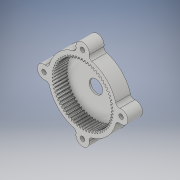
# Autodesk Inventor part: RushGears_AP214_F3264A
Saved by Autodesk Inventor 2019 (Build 230136000, 136)
## iProperties
Company: Microsoft
Created: 2015-06-23
Part Number: RushGears_AP214_F3264A
Material: Generic
Description: STEP AP214
Document SubType Name: Modeling
Designer: test
Density: 1 g/cm^3
Appearance: Default
Sending System: SolidWorks 2010
Preprocessor: SwSTEP 2.0
Title: 698691a11791bb78f6e835ded6c04318_ap214.step
Author: Solidworks
Revision Number: ANY
Autodesk Inventor part; units mm, degrees
(part 1 of 4)
ref_plane "YZ Plane" through (0, 0, 0) normal (1, 0, 0) x (0, 1, 0)
ref_plane "Work Plane2" through (20.4322, -12.3376, 4.826) normal (0, 0, 1) x (0.8768168, -0.4808246, 0)
ref_plane "Work Plane1" through (20.4322, -12.3376, 27.051) normal (0, 0, 1) x (0.8768168, -0.4808246, 0)
sketch "Sketch2" plane through (20.4322, -12.3376, 27.051) normal (0, 0, 1) x (0.8768168, -0.4808246, 0)
  arc A0 (1.0525, 9.1239) -> (0.8407, 9.7461) centre (-23.8475, 0.9936) ccw projected
  arc A1 (0.8407, 9.7461) -> (-0.8407, 9.7461) centre (0, 0) ccw projected
  arc A2 (-1.1493, 9.9373) -> (-0.8407, 9.7461) centre (-0.8668, 10.0487) ccw projected
  arc A3 (-1.1493, 9.9373) -> (-1.1833, 10.0231) centre (-23.8475, 0.9936) ccw projected
  arc A4 (-1.0894, 10.3738) -> (-1.1833, 10.0231) centre (-0.9012, 10.1355) ccw projected
  arc A5 (-1.0894, 10.3738) -> (0.1357, 11.5254) centre (-7.1521, 18.0509) ccw projected
  arc A6 (0.1357, 11.5254) -> (-0.1361, 12.1238) centre (-23.8475, 0.9936) ccw projected
  arc A7 (-0.1361, 12.1238) -> (-1.8093, 11.959) centre (-0.0174, 2.3422) ccw projected
  arc A8 (-2.1353, 12.1191) -> (-1.8093, 11.959) centre (-1.865, 12.2576) ccw projected
  arc A9 (-2.1353, 12.1191) -> (-2.1775, 12.2011) centre (-23.8475, 0.9936) ccw projected
  arc A10 (-2.1184, 12.5594) -> (-2.1775, 12.2011) centre (-1.9077, 12.3406) ccw projected
  arc A11 (-2.1184, 12.5594) -> (-1.0121, 13.8254) centre (-8.9044, 19.6052) ccw projected
  arc A12 (-1.0121, 13.8254) -> (-1.3412, 14.3943) centre (-23.8475, 0.9936) ccw projected
  arc A13 (-1.3412, 14.3943) -> (-2.9903, 14.0663) centre (-0.2644, 4.6715) ccw projected
  arc A14 (-3.3303, 14.1937) -> (-2.9903, 14.0663) centre (-3.0749, 14.358) ccw projected
  arc A15 (-3.3303, 14.1937) -> (-3.3804, 14.2712) centre (-23.8475, 0.9936) ccw projected
  arc A16 (-3.3567, 14.6335) -> (-3.3804, 14.2712) centre (-3.1256, 14.4365) ccw projected
  arc A17 (-3.3567, 14.6335) -> (-2.3798, 16.0019) centre (-10.8006, 20.9803) ccw projected
  arc A18 (-2.3798, 16.0019) -> (-2.7631, 16.5358) centre (-23.8475, 0.9936) ccw projected
  arc A19 (-2.7631, 16.5358) -> (-4.3721, 16.0477) centre (-0.7385, 6.9653) ccw projected
  arc A20 (-4.7229, 16.1411) -> (-4.3721, 16.0477) centre (-4.4849, 16.3297) ccw projected
  arc A21 (-4.7229, 16.1411) -> (-4.7804, 16.2134) centre (-23.8475, 0.9936) ccw projected
  arc A22 (-4.7923, 16.5763) -> (-4.7804, 16.2134) centre (-4.543, 16.4028) ccw projected
  arc A23 (-4.7923, 16.5763) -> (-3.9543, 18.0339) centre (-12.8224, 22.1628) ccw projected
  arc A24 (-3.9543, 18.0339) -> (-4.3881, 18.5276) centre (-23.8475, 0.9936) ccw projected
  arc A25 (-4.3881, 18.5276) -> (-5.9414, 17.8842) centre (-1.4351, 9.2017) ccw projected
  arc A26 (-6.2997, 17.9427) -> (-5.9414, 17.8842) centre (-6.0813, 18.1537) ccw projected
  arc A27 (-6.2997, 17.9427) -> (-6.364, 18.009) centre (-23.8475, 0.9936) ccw projected
  arc A28 (-6.4114, 18.369) -> (-6.364, 18.009) centre (-6.1463, 18.2208) ccw projected
  arc A29 (-6.4114, 18.369) -> (-5.7203, 19.9017) centre (-14.9505, 23.1415) ccw projected
  arc A30 (-5.7203, 19.9017) -> (-6.2004, 20.3505) centre (-23.8475, 0.9936) ccw projected
  arc A31 (-6.2004, 20.3505) -> (-7.6832, 19.5579) centre (-2.3475, 11.359) ccw projected
  arc A32 (-8.0455, 19.5811) -> (-7.6832, 19.5579) centre (-7.8488, 19.8125) ccw projected
  arc A33 (-8.0455, 19.5811) -> (-8.116, 19.6407) centre (-23.8475, 0.9936) ccw projected
  arc A34 (-8.1985, 19.9943) -> (-8.116, 19.6407) centre (-7.9201, 19.8729) ccw projected
  arc A35 (-8.1985, 19.9943) -> (-7.6609, 21.5874) centre (-17.1642, 23.907) ccw projected
  arc A36 (-7.6609, 21.5874) -> (-8.1827, 21.987) centre (-23.8475, 0.9936) ccw projected
  arc A37 (-8.1827, 21.987) -> (-9.5807, 21.0529) centre (-3.467, 13.4164) ccw projected
  arc A38 (-9.9435, 21.0405) -> (-9.5807, 21.0529) centre (-9.7705, 21.29) ccw projected
  arc A39 (-9.9435, 21.0405) -> (-10.0195, 21.0929) centre (-23.8475, 0.9936) ccw projected
  arc A40 (-10.1362, 21.4367) -> (-10.0195, 21.0929) centre (-9.8473, 21.3431) ccw projected
  arc A41 (-10.1362, 21.4367) -> (-9.7574, 23.0748) centre (-19.4423, 24.4517) ccw projected
  arc A42 (-9.7574, 23.0748) -> (-10.3158, 23.4214) centre (-23.8475, 0.9936) ccw projected
  arc A43 (-10.3158, 23.4214) -> (-11.6155, 22.3547) centre (-4.7828, 15.3542) ccw projected
  arc A44 (-11.9754, 22.3068) -> (-11.6155, 22.3547) centre (-11.8276, 22.5721) ccw projected
  arc A45 (-11.9754, 22.3068) -> (-12.0561, 22.3515) centre (-23.8475, 0.9936) ccw projected
  arc A46 (-12.206, 22.6822) -> (-12.0561, 22.3515) centre (-11.9093, 22.6174) ccw projected
  arc A47 (-12.206, 22.6822) -> (-11.9896, 24.3495) centre (-21.7628, 24.7705) ccw projected
  arc A48 (-11.9896, 24.3495) -> (-12.5793, 24.6397) centre (-23.8475, 0.9936) ccw projected
  arc A49 (-12.5793, 24.6397) -> (-13.7682, 23.4508) centre (-6.2822, 17.1537) ccw projected
  arc A50 (-14.1217, 23.3678) -> (-13.7682, 23.4508) centre (-14.0006, 23.6463) ccw projected
  arc A51 (-14.1217, 23.3678) -> (-14.2064, 23.4044) centre (-23.8475, 0.9936) ccw projected
  arc A52 (-14.388, 23.7188) -> (-14.2064, 23.4044) centre (-14.0863, 23.6834) ccw projected
  arc A53 (-14.388, 23.7188) -> (-14.336, 25.3994) centre (-24.1034, 24.8604) ccw projected
  arc A54 (-14.336, 25.3994) -> (-14.9513, 25.6303) centre (-23.8475, 0.9936) ccw projected
  arc A55 (-14.9513, 25.6303) -> (-16.0179, 24.3306) centre (-7.9508, 18.7976) ccw projected
  arc A56 (-16.3615, 24.2134) -> (-16.0179, 24.3306) centre (-16.2684, 24.5024) ccw projected
  arc A57 (-16.3615, 24.2134) -> (-16.4494, 24.2415) centre (-23.8475, 0.9936) ccw projected
  arc A58 (-16.661, 24.5366) -> (-16.4494, 24.2415) centre (-16.3573, 24.5309) ccw projected
  arc A59 (-16.661, 24.5366) -> (-16.774, 26.2141) centre (-26.4415, 24.7204) ccw projected
  arc A60 (-16.774, 26.2141) -> (-17.409, 26.3837) centre (-23.8475, 0.9936) ccw projected
  arc A61 (-17.409, 26.3837) -> (-18.3431, 24.9857) centre (-9.7724, 20.27) ccw projected
  arc A62 (-18.6735, 24.8353) -> (-18.3431, 24.9857) centre (-18.6091, 25.1321) ccw projected
  arc A63 (-18.6735, 24.8353) -> (-18.7637, 24.8547) centre (-23.8475, 0.9936) ccw projected
  arc A64 (-19.0032, 25.1276) -> (-18.7637, 24.8547) centre (-18.7005, 25.1517) ccw projected
  arc A65 (-19.0032, 25.1276) -> (-19.2801, 26.786) centre (-28.7547, 24.3519) ccw projected
  arc A66 (-19.2801, 26.786) -> (-19.9286, 26.8925) centre (-23.8475, 0.9936) ccw projected
  arc A67 (-19.9286, 26.8925) -> (-20.7212, 25.4097) centre (-11.7296, 21.5568) ccw projected
  arc A68 (-21.0353, 25.2276) -> (-20.7212, 25.4097) centre (-21.0003, 25.5293) ccw projected
  arc A69 (-21.0353, 25.2276) -> (-21.127, 25.2381) centre (-23.8475, 0.9936) ccw projected
  arc A70 (-21.3921, 25.4863) -> (-21.127, 25.2381) centre (-21.0932, 25.5399) ccw projected
  arc A71 (-21.3921, 25.4863) -> (-21.8302, 27.1095) centre (-31.0205, 23.7584) ccw projected
  arc A72 (-21.8302, 27.1095) -> (-22.486, 27.1519) centre (-23.8475, 0.9936) ccw projected
  arc A73 (-22.486, 27.1519) -> (-23.1295, 25.5986) centre (-13.8035, 22.6456) ccw projected
  arc A74 (-23.4242, 25.3866) -> (-23.1295, 25.5986) centre (-23.419, 25.6902) ccw projected
  arc A75 (-23.4242, 25.3866) -> (-23.5165, 25.388) centre (-23.8475, 0.9936) ccw projected
  arc A76 (-23.8046, 25.609) -> (-23.5165, 25.388) centre (-23.5124, 25.6917) ccw projected
  arc A77 (-23.8046, 25.609) -> (-24.3997, 27.1815) centre (-33.2174, 22.9457) ccw projected
  arc A78 (-24.3997, 27.1815) -> (-25.0566, 27.1594) centre (-23.8475, 0.9936) ccw projected
  arc A79 (-25.0566, 27.1594) -> (-25.5446, 25.5505) centre (-15.9742, 23.5258) ccw projected
  arc A80 (-25.8172, 25.3106) -> (-25.5446, 25.5505) centre (-25.8417, 25.6133) ccw projected
  arc A81 (-25.8172, 25.3106) -> (-25.9092, 25.303) centre (-23.8475, 0.9936) ccw projected
  arc A82 (-26.2175, 25.4947) -> (-25.9092, 25.303) centre (-25.9348, 25.6056) ccw projected
  arc A83 (-26.2175, 25.4947) -> (-26.9639, 27.0013) centre (-35.3239, 21.9216) ccw projected
  arc A84 (-26.9639, 27.0013) -> (-27.6154, 26.9149) centre (-23.8475, 0.9936) ccw projected
  arc A85 (-27.6154, 26.9149) -> (-27.9434, 25.2659) centre (-18.2206, 24.189) ccw projected
  arc A86 (-28.1912, 25.0005) -> (-27.9434, 25.2659) centre (-28.2453, 25.2993) ccw projected
  arc A87 (-28.1912, 25.0005) -> (-28.282, 24.9839) centre (-23.8475, 0.9936) ccw projected
  arc A88 (-28.6077, 25.1444) -> (-28.282, 24.9839) centre (-28.3372, 25.2825) ccw projected
  arc A89 (-28.6077, 25.1444) -> (-29.4981, 26.5706) centre (-37.32, 20.6959) ccw projected
  arc A90 (-29.4981, 26.5706) -> (-30.138, 26.4207) centre (-23.8475, 0.9936) ccw projected
  arc A91 (-30.138, 26.4207) -> (-30.3028, 24.7475) centre (-20.5213, 24.6288) ccw projected
  arc A92 (-30.5234, 24.4591) -> (-30.3028, 24.7475) centre (-30.6065, 24.7512) ccw projected
  arc A93 (-30.5234, 24.4591) -> (-30.6121, 24.4337) centre (-23.8475, 0.9936) ccw projected
  arc A94 (-30.9519, 24.5615) -> (-30.6121, 24.4337) centre (-30.6963, 24.7255) ccw projected
  arc A95 (-30.9519, 24.5615) -> (-31.9779, 25.8935) centre (-39.1863, 19.2805) ccw projected
  arc A96 (-31.9779, 25.8935) -> (-32.6, 25.6817) centre (-23.8475, 0.9936) ccw projected
  arc A97 (-32.6, 25.6817) -> (-32.6, 24.0004) centre (-22.8539, 24.8411) ccw projected
  arc A98 (-32.7913, 23.6917) -> (-32.6, 24.0004) centre (-32.9026, 23.9743) ccw projected
  arc A99 (-32.7913, 23.6917) -> (-32.8771, 23.6578) centre (-23.8475, 0.9936) ccw projected
  arc A100 (-33.2278, 23.7517) -> (-32.8771, 23.6578) centre (-32.9895, 23.9399) ccw projected
  arc A101 (-33.2278, 23.7517) -> (-34.3794, 24.9767) centre (-40.9048, 17.689) ccw projected
  arc A102 (-34.3794, 24.9767) -> (-34.9778, 24.7049) centre (-23.8475, 0.9936) ccw projected
  arc A103 (-34.9778, 24.7049) -> (-34.813, 23.0317) centre (-25.1962, 24.8236) ccw projected
  arc A104 (-34.973, 22.7058) -> (-34.813, 23.0317) centre (-35.1115, 22.9761) ccw projected
  arc A105 (-34.973, 22.7058) -> (-35.0551, 22.6636) centre (-23.8475, 0.9936) ccw projected
  arc A106 (-35.4133, 22.7227) -> (-35.0551, 22.6636) centre (-35.1946, 22.9333) ccw projected
  arc A107 (-35.4133, 22.7227) -> (-36.6794, 23.8289) centre (-42.4591, 15.9367) ccw projected
  arc A108 (-36.6794, 23.8289) -> (-37.2483, 23.4998) centre (-23.8475, 0.9936) ccw projected
  arc A109 (-37.2483, 23.4998) -> (-36.9203, 21.8508) centre (-27.5255, 24.5767) ccw projected
  arc A110 (-37.0476, 21.5108) -> (-36.9203, 21.8508) centre (-37.2119, 21.7662) ccw projected
  arc A111 (-37.0476, 21.5108) -> (-37.1251, 21.4607) centre (-23.8475, 0.9936) ccw projected
  arc A112 (-37.4874, 21.4844) -> (-37.1251, 21.4607) centre (-37.2904, 21.7155) ccw projected
  arc A113 (-37.4874, 21.4844) -> (-38.8559, 22.4612) centre (-43.8342, 14.0405) ccw projected
  arc A114 (-38.8559, 22.4612) -> (-39.3898, 22.0779) centre (-23.8475, 0.9936) ccw projected
  arc A115 (-39.3898, 22.0779) -> (-38.9017, 20.469) centre (-29.8193, 24.1026) ccw projected
  arc A116 (-38.9951, 20.1181) -> (-38.9017, 20.469) centre (-39.1836, 20.3562) ccw projected
  arc A117 (-38.9951, 20.1181) -> (-39.0673, 20.0607) centre (-23.8475, 0.9936) ccw projected
  arc A118 (-39.4302, 20.0488) -> (-39.0673, 20.0607) centre (-39.2568, 20.2981) ccw projected
  arc A119 (-39.4302, 20.0488) -> (-40.8878, 20.8868) centre (-45.0168, 12.0186) ccw projected
  arc A120 (-40.8878, 20.8868) -> (-41.3815, 20.453) centre (-23.8475, 0.9936) ccw projected
  arc A121 (-41.3815, 20.453) -> (-40.7381, 18.8997) centre (-32.0556, 23.406) ccw projected
  arc A122 (-40.7967, 18.5413) -> (-40.7381, 18.8997) centre (-41.0077, 18.7598) ccw projected
  arc A123 (-40.7967, 18.5413) -> (-40.8629, 18.4771) centre (-23.8475, 0.9936) ccw projected
  arc A124 (-41.2229, 18.4296) -> (-40.8629, 18.4771) centre (-41.0747, 18.6947) ccw projected
  arc A125 (-41.2229, 18.4296) -> (-42.7556, 19.1208) centre (-45.9955, 9.8906) ccw projected
  arc A126 (-42.7556, 19.1208) -> (-43.2045, 18.6407) centre (-23.8475, 0.9936) ccw projected
  arc A127 (-43.2045, 18.6407) -> (-42.4119, 17.1579) centre (-34.2129, 22.4935) ccw projected
  arc A128 (-42.4351, 16.7955) -> (-42.4119, 17.1579) centre (-42.6664, 16.9922) ccw projected
  arc A129 (-42.4351, 16.7955) -> (-42.4947, 16.7251) centre (-23.8475, 0.9936) ccw projected
  arc A130 (-42.8483, 16.6426) -> (-42.4947, 16.7251) centre (-42.7268, 16.9209) ccw projected
  arc A131 (-42.8483, 16.6426) -> (-44.4414, 17.1802) centre (-46.7609, 7.6769) ccw projected
  arc A132 (-44.4414, 17.1802) -> (-44.841, 16.6584) centre (-23.8475, 0.9936) ccw projected
  arc A133 (-44.841, 16.6584) -> (-43.9069, 15.2604) centre (-36.2704, 21.374) ccw projected
  arc A134 (-43.8944, 14.8975) -> (-43.9069, 15.2604) centre (-44.144, 15.0706) ccw projected
  arc A135 (-43.8944, 14.8975) -> (-43.9469, 14.8216) centre (-23.8475, 0.9936) ccw projected
  arc A136 (-44.2907, 14.7048) -> (-43.9469, 14.8216) centre (-44.1971, 14.9937) ccw projected
  arc A137 (-44.2907, 14.7048) -> (-45.9288, 15.0837) centre (-47.3057, 5.3988) ccw projected
  arc A138 (-45.9288, 15.0837) -> (-46.2753, 14.5252) centre (-23.8475, 0.9936) ccw projected
  arc A139 (-46.2753, 14.5252) -> (-45.2087, 13.2255) centre (-38.2082, 20.0582) ccw projected
  arc A140 (-45.1607, 12.8656) -> (-45.2087, 13.2255) centre (-45.426, 13.0134) ccw projected
  arc A141 (-45.1607, 12.8656) -> (-45.2055, 12.7849) centre (-23.8475, 0.9936) ccw projected
  arc A142 (-45.5362, 12.635) -> (-45.2055, 12.7849) centre (-45.4713, 12.9317) ccw projected
  arc A143 (-45.5362, 12.635) -> (-47.2035, 12.8515) centre (-47.6245, 3.0783) ccw projected
  arc A144 (-47.2035, 12.8515) -> (-47.4937, 12.2618) centre (-23.8475, 0.9936) ccw projected
  arc A145 (-47.4937, 12.2618) -> (-46.3048, 11.0729) centre (-40.0077, 18.5588) ccw projected
  arc A146 (-46.2217, 10.7194) -> (-46.3048, 11.0729) centre (-46.5003, 10.8405) ccw projected
  arc A147 (-46.2217, 10.7194) -> (-46.2584, 10.6347) centre (-23.8475, 0.9936) ccw projected
  arc A148 (-46.5728, 10.4531) -> (-46.2584, 10.6347) centre (-46.5373, 10.7547) ccw projected
  arc A149 (-46.5728, 10.4531) -> (-48.2533, 10.5051) centre (-47.7143, 0.7377) ccw projected
  arc A150 (-48.2533, 10.5051) -> (-48.4843, 9.8898) centre (-23.8475, 0.9936) ccw projected
  arc A151 (-48.4843, 9.8898) -> (-47.1846, 8.8231) centre (-41.6516, 16.8903) ccw projected
  arc A152 (-47.0673, 8.4795) -> (-47.1846, 8.8231) centre (-47.3563, 8.5727) ccw projected
  arc A153 (-47.0673, 8.4795) -> (-47.0955, 8.3916) centre (-23.8475, 0.9936) ccw projected
  arc A154 (-47.3906, 8.1801) -> (-47.0955, 8.3916) centre (-47.3848, 8.4837) ccw projected
  arc A155 (-47.3906, 8.1801) -> (-49.0681, 8.0671) centre (-47.5743, -1.6005) ccw projected
  arc A156 (-49.0681, 8.0671) -> (-49.2376, 7.4321) centre (-23.8475, 0.9936) ccw projected
  arc A157 (-49.2376, 7.4321) -> (-47.8396, 6.498) centre (-43.124, 15.0686) ccw projected
  arc A158 (-47.6893, 6.1675) -> (-47.8396, 6.498) centre (-47.986, 6.2319) ccw projected
  arc A159 (-47.6893, 6.1675) -> (-47.7087, 6.0773) centre (-23.8475, 0.9936) ccw projected
  arc A160 (-47.9816, 5.8379) -> (-47.7087, 6.0773) centre (-48.0057, 6.1406) ccw projected
  arc A161 (-47.9816, 5.8379) -> (-49.64, 5.561) centre (-47.2058, -3.9136) ccw projected
  arc A162 (-49.64, 5.561) -> (-49.7464, 4.9124) centre (-23.8475, 0.9936) ccw projected
  arc A163 (-49.7464, 4.9124) -> (-48.2636, 4.1199) centre (-44.4108, 13.1114) ccw projected
  arc A164 (-48.0816, 3.8057) -> (-48.2636, 4.1199) centre (-48.3833, 3.8407) ccw projected
  arc A165 (-48.0816, 3.8057) -> (-48.092, 3.714) centre (-23.8475, 0.9936) ccw projected
  arc A166 (-48.3402, 3.449) -> (-48.092, 3.714) centre (-48.3938, 3.7479) ccw projected
  arc A167 (-48.3402, 3.449) -> (-49.9635, 3.0109) centre (-46.6123, -6.1795) ccw projected
  arc A168 (-49.9635, 3.0109) -> (-50.0058, 2.355) centre (-23.8475, 0.9936) ccw projected
  arc A169 (-50.0058, 2.355) -> (-48.4525, 1.7116) centre (-45.4995, 11.0375) ccw projected
  arc A170 (-48.2405, 1.4168) -> (-48.4525, 1.7116) centre (-48.5442, 1.4221) ccw projected
  arc A171 (-48.2405, 1.4168) -> (-48.242, 1.3246) centre (-23.8475, 0.9936) ccw projected
  arc A172 (-48.4629, 1.0365) -> (-48.242, 1.3246) centre (-48.5456, 1.3287) ccw projected
  arc A173 (-48.4629, 1.0365) -> (-50.0354, 0.4414) centre (-45.7996, -8.3763) ccw projected
  arc A174 (-50.0354, 0.4414) -> (-50.0133, -0.2155) centre (-23.8475, 0.9936) ccw projected
  arc A175 (-50.0133, -0.2155) -> (-48.4044, -0.7036) centre (-46.3797, 8.8669) ccw projected
  arc A176 (-48.1646, -0.9762) -> (-48.4044, -0.7036) centre (-48.4673, -1.0007) ccw projected
  arc A177 (-48.1646, -0.9762) -> (-48.1569, -1.0681) centre (-23.8475, 0.9936) ccw projected
  arc A178 (-48.3486, -1.3765) -> (-48.1569, -1.0681) centre (-48.4595, -1.0938) ccw projected
  arc A179 (-48.3486, -1.3765) -> (-49.8552, -2.1228) centre (-44.7755, -10.4829) ccw projected
  arc A180 (-49.8552, -2.1228) -> (-49.7688, -2.7744) centre (-23.8475, 0.9936) ccw projected
  arc A181 (-49.7688, -2.7744) -> (-48.1198, -3.1024) centre (-47.043, 6.6204) ccw projected
  arc A182 (-47.8544, -3.3502) -> (-48.1198, -3.1024) centre (-48.1532, -3.4042) ccw projected
  arc A183 (-47.8544, -3.3502) -> (-47.8378, -3.4409) centre (-23.8475, 0.9936) ccw projected
  arc A184 (-47.9983, -3.7666) -> (-47.8378, -3.4409) centre (-48.1364, -3.4961) ccw projected
  arc A185 (-47.9983, -3.7666) -> (-49.4245, -4.657) centre (-43.5499, -12.4789) ccw projected
  arc A186 (-49.4245, -4.657) -> (-49.2747, -5.297) centre (-23.8475, 0.9936) ccw projected
  arc A187 (-49.2747, -5.297) -> (-47.6015, -5.4618) centre (-47.4828, 4.3198) ccw projected
  arc A188 (-47.313, -5.6823) -> (-47.6015, -5.4618) centre (-47.6051, -5.7654) ccw projected
  arc A189 (-47.313, -5.6823) -> (-47.2876, -5.771) centre (-23.8475, 0.9936) ccw projected
  arc A190 (-47.4155, -6.1109) -> (-47.2876, -5.771) centre (-47.5794, -5.8552) ccw projected
  arc A191 (-47.4155, -6.1109) -> (-48.7475, -7.1368) centre (-42.1345, -14.3452) ccw projected
  arc A192 (-48.7475, -7.1368) -> (-48.5357, -7.759) centre (-23.8475, 0.9936) ccw projected
  arc A193 (-48.5357, -7.759) -> (-46.8543, -7.759) centre (-47.695, 1.9871) ccw projected
  arc A194 (-46.5457, -7.9502) -> (-46.8543, -7.759) centre (-46.8282, -8.0615) ccw projected
  arc A195 (-46.5457, -7.9502) -> (-46.5117, -8.036) centre (-23.8475, 0.9936) ccw projected
  arc A196 (-46.6056, -8.3867) -> (-46.5117, -8.036) centre (-46.7938, -8.1484) ccw projected
  arc A197 (-46.6056, -8.3867) -> (-47.8307, -9.5383) centre (-40.543, -16.0638) ccw projected
  arc A198 (-47.8307, -9.5383) -> (-47.5589, -10.1367) centre (-23.8475, 0.9936) ccw projected
  arc A199 (-47.5589, -10.1367) -> (-45.8857, -9.9719) centre (-47.6776, -0.3551) ccw projected
  arc A200 (-45.5598, -10.132) -> (-45.8857, -9.9719) centre (-45.83, -10.2704) ccw projected
  arc A201 (-45.5598, -10.132) -> (-45.5175, -10.214) centre (-23.8475, 0.9936) ccw projected
  arc A202 (-45.5766, -10.5722) -> (-45.5175, -10.214) centre (-45.7873, -10.3535) ccw projected
  arc A203 (-45.5766, -10.5722) -> (-46.6829, -11.8383) centre (-38.7907, -17.6181) ccw projected
  arc A204 (-46.6829, -11.8383) -> (-46.3538, -12.4072) centre (-23.8475, 0.9936) ccw projected
  arc A205 (-46.3538, -12.4072) -> (-44.7047, -12.0792) centre (-47.4306, -2.6844) ccw projected
  arc A206 (-44.3647, -12.2066) -> (-44.7047, -12.0792) centre (-44.6201, -12.3709) ccw projected
  arc A207 (-44.3647, -12.2066) -> (-44.3146, -12.2841) centre (-23.8475, 0.9936) ccw projected
  arc A208 (-44.3383, -12.6464) -> (-44.3146, -12.2841) centre (-44.5694, -12.4493) ccw projected
  arc A209 (-44.3383, -12.6464) -> (-45.3152, -14.0148) centre (-36.8944, -18.9931) ccw projected
  arc A210 (-45.3152, -14.0148) -> (-44.9319, -14.5487) centre (-23.8475, 0.9936) ccw projected
  arc A211 (-44.9319, -14.5487) -> (-43.323, -14.0606) centre (-46.9566, -4.9782) ccw projected
  arc A212 (-42.9721, -14.154) -> (-43.323, -14.0606) centre (-43.2101, -14.3426) ccw projected
  arc A213 (-42.9721, -14.154) -> (-42.9147, -14.2263) centre (-23.8475, 0.9936) ccw projected
  arc A214 (-42.9027, -14.5891) -> (-42.9147, -14.2263) centre (-43.152, -14.4157) ccw projected
  arc A215 (-42.9027, -14.5891) -> (-43.7407, -16.0467) centre (-34.8726, -20.1757) ccw projected
  arc A216 (-43.7407, -16.0467) -> (-43.307, -16.5405) centre (-23.8475, 0.9936) ccw projected
  arc A217 (-43.307, -16.5405) -> (-41.7536, -15.8971) centre (-46.2599, -7.2146) ccw projected
  arc A218 (-41.3953, -15.9556) -> (-41.7536, -15.8971) centre (-41.6137, -16.1666) ccw projected
  arc A219 (-41.3953, -15.9556) -> (-41.331, -16.0219) centre (-23.8475, 0.9936) ccw projected
  arc A220 (-41.2836, -16.3819) -> (-41.331, -16.0219) centre (-41.5487, -16.2337) ccw projected
  arc A221 (-41.2836, -16.3819) -> (-41.9747, -17.9146) centre (-32.7445, -21.1544) ccw projected
  arc A222 (-41.9747, -17.9146) -> (-41.4946, -18.3634) centre (-23.8475, 0.9936) ccw projected
  arc A223 (-41.4946, -18.3634) -> (-40.0118, -17.5708) centre (-45.3475, -9.3718) ccw projected
  arc A224 (-39.6495, -17.594) -> (-40.0118, -17.5708) centre (-39.8462, -17.8254) ccw projected
  arc A225 (-39.6495, -17.594) -> (-39.579, -17.6536) centre (-23.8475, 0.9936) ccw projected
  arc A226 (-39.4965, -18.0072) -> (-39.579, -17.6536) centre (-39.7749, -17.8858) ccw projected
  arc A227 (-39.4965, -18.0072) -> (-40.0341, -19.6003) centre (-30.5308, -21.9198) ccw projected
  arc A228 (-40.0341, -19.6003) -> (-39.5123, -19.9999) centre (-23.8475, 0.9936) ccw projected
  arc A229 (-39.5123, -19.9999) -> (-38.1143, -19.0658) centre (-44.228, -11.4293) ccw projected
  arc A230 (-37.7515, -19.0534) -> (-38.1143, -19.0658) centre (-37.9245, -19.3029) ccw projected
  arc A231 (-37.7515, -19.0534) -> (-37.6756, -19.1058) centre (-23.8475, 0.9936) ccw projected
  arc A232 (-37.5588, -19.4496) -> (-37.6756, -19.1058) centre (-37.8477, -19.356) ccw projected
  arc A233 (-37.5588, -19.4496) -> (-37.9376, -21.0877) centre (-28.2527, -22.4646) ccw projected
  arc A234 (-37.9376, -21.0877) -> (-37.3792, -21.4343) centre (-23.8475, 0.9936) ccw projected
  arc A235 (-37.3792, -21.4343) -> (-36.0795, -20.3676) centre (-42.9122, -13.3671) ccw projected
  arc A236 (-35.7196, -20.3197) -> (-36.0795, -20.3676) centre (-35.8674, -20.585) ccw projected
  arc A237 (-35.7196, -20.3197) -> (-35.6389, -20.3644) centre (-23.8475, 0.9936) ccw projected
  arc A238 (-35.489, -20.6951) -> (-35.6389, -20.3644) centre (-35.7857, -20.6303) ccw projected
  arc A239 (-35.489, -20.6951) -> (-35.7054, -22.3624) centre (-25.9322, -22.7834) ccw projected
  arc A240 (-35.7054, -22.3624) -> (-35.1157, -22.6526) centre (-23.8475, 0.9936) ccw projected
  arc A241 (-35.1157, -22.6526) -> (-33.9268, -21.4637) centre (-41.4128, -15.1666) ccw projected
  arc A242 (-33.5734, -21.3807) -> (-33.9268, -21.4637) centre (-33.6944, -21.6592) ccw projected
  arc A243 (-33.5734, -21.3807) -> (-33.4887, -21.4173) centre (-23.8475, 0.9936) ccw projected
  arc A244 (-33.3071, -21.7317) -> (-33.4887, -21.4173) centre (-33.6087, -21.6963) ccw projected
  arc A245 (-33.3071, -21.7317) -> (-33.359, -23.4123) centre (-23.5916, -22.8733) ccw projected
  arc A246 (-33.359, -23.4123) -> (-32.7437, -23.6432) centre (-23.8475, 0.9936) ccw projected
  arc A247 (-32.7437, -23.6432) -> (-31.6771, -22.3435) centre (-39.7442, -16.8105) ccw projected
  arc A248 (-31.3335, -22.2263) -> (-31.6771, -22.3435) centre (-31.4266, -22.5153) ccw projected
  arc A249 (-31.3335, -22.2263) -> (-31.2456, -22.2544) centre (-23.8475, 0.9936) ccw projected
  arc A250 (-31.034, -22.5495) -> (-31.2456, -22.2544) centre (-31.3377, -22.5438) ccw projected
  arc A251 (-31.034, -22.5495) -> (-30.921, -24.227) centre (-21.2535, -22.7333) ccw projected
  arc A252 (-30.921, -24.227) -> (-30.2861, -24.3966) centre (-23.8475, 0.9936) ccw projected
  arc A253 (-30.2861, -24.3966) -> (-29.352, -22.9986) centre (-37.9226, -18.2829) ccw projected
  arc A254 (-29.0215, -22.8482) -> (-29.352, -22.9986) centre (-29.0859, -23.145) ccw projected
  arc A255 (-29.0215, -22.8482) -> (-28.9313, -22.8676) centre (-23.8475, 0.9936) ccw projected
  arc A256 (-28.6918, -23.1405) -> (-28.9313, -22.8676) centre (-28.9945, -23.1646) ccw projected
  arc A257 (-28.6918, -23.1405) -> (-28.4149, -24.7989) centre (-18.9403, -22.3648) ccw projected
  arc A258 (-28.4149, -24.7989) -> (-27.7664, -24.9054) centre (-23.8475, 0.9936) ccw projected
  arc A259 (-27.7664, -24.9054) -> (-26.9738, -23.4226) centre (-35.9654, -19.5697) ccw projected
  arc A260 (-26.6597, -23.2405) -> (-26.9738, -23.4226) centre (-26.6947, -23.5422) ccw projected
  arc A261 (-26.6597, -23.2405) -> (-26.568, -23.251) centre (-23.8475, 0.9936) ccw projected
  arc A262 (-26.3029, -23.4991) -> (-26.568, -23.251) centre (-26.6018, -23.5528) ccw projected
  arc A263 (-26.3029, -23.4991) -> (-25.8648, -25.1224) centre (-16.6745, -21.7713) ccw projected
  arc A264 (-25.8648, -25.1224) -> (-25.209, -25.1648) centre (-23.8475, 0.9936) ccw projected
  arc A265 (-25.209, -25.1648) -> (-24.5656, -23.6114) centre (-33.8915, -20.6584) ccw projected
  arc A266 (-24.2708, -23.3995) -> (-24.5656, -23.6114) centre (-24.276, -23.7031) ccw projected
  arc A267 (-24.2708, -23.3995) -> (-24.1785, -23.4009) centre (-23.8475, 0.9936) ccw projected
  arc A268 (-23.8904, -23.6219) -> (-24.1785, -23.4009) centre (-24.1826, -23.7046) ccw projected
  arc A269 (-23.8904, -23.6219) -> (-23.2953, -25.1944) centre (-14.4777, -20.9586) ccw projected
  arc A270 (-23.2953, -25.1944) -> (-22.6385, -25.1723) centre (-23.8475, 0.9936) ccw projected
  arc A271 (-22.6385, -25.1723) -> (-22.1504, -23.5633) centre (-31.7208, -21.5387) ccw projected
  arc A272 (-21.8778, -23.3235) -> (-22.1504, -23.5633) centre (-21.8533, -23.6262) ccw projected
  arc A273 (-21.8778, -23.3235) -> (-21.7858, -23.3159) centre (-23.8475, 0.9936) ccw projected
  arc A274 (-21.4775, -23.5076) -> (-21.7858, -23.3159) centre (-21.7602, -23.6185) ccw projected
  arc A275 (-21.4775, -23.5076) -> (-20.7311, -25.0141) centre (-12.3711, -19.9345) ccw projected
  arc A276 (-20.7311, -25.0141) -> (-20.0796, -24.9278) centre (-23.8475, 0.9936) ccw projected
  arc A277 (-20.0796, -24.9278) -> (-19.7516, -23.2787) centre (-29.4744, -22.2019) ccw projected
  arc A278 (-19.5038, -23.0133) -> (-19.7516, -23.2787) centre (-19.4497, -23.3122) ccw projected
  arc A279 (-19.5038, -23.0133) -> (-19.413, -22.9967) centre (-23.8475, 0.9936) ccw projected
  arc A280 (-19.0873, -23.1573) -> (-19.413, -22.9967) centre (-19.3578, -23.2954) ccw projected
  arc A281 (-19.0873, -23.1573) -> (-18.1969, -24.5835) centre (-10.375, -18.7088) ccw projected
  arc A282 (-18.1969, -24.5835) -> (-17.557, -24.4336) centre (-23.8475, 0.9936) ccw projected
  arc A283 (-17.557, -24.4336) -> (-17.3922, -22.7604) centre (-27.1737, -22.6417) ccw projected
  arc A284 (-17.1716, -22.472) -> (-17.3922, -22.7604) centre (-17.0885, -22.7641) ccw projected
  arc A285 (-17.1716, -22.472) -> (-17.0829, -22.4466) centre (-23.8475, 0.9936) ccw projected
  arc A286 (-16.7431, -22.5744) -> (-17.0829, -22.4466) centre (-16.9987, -22.7383) ccw projected
  arc A287 (-16.7431, -22.5744) -> (-15.7171, -23.9064) centre (-8.5087, -17.2934) ccw projected
  arc A288 (-15.7171, -23.9064) -> (-15.095, -23.6946) centre (-23.8475, 0.9936) ccw projected
  arc A289 (-15.095, -23.6946) -> (-15.095, -22.0133) centre (-24.8411, -22.8539) ccw projected
  arc A290 (-14.9037, -21.7046) -> (-15.095, -22.0133) centre (-14.7924, -21.9872) ccw projected
  arc A291 (-14.9037, -21.7046) -> (-14.818, -21.6706) centre (-23.8475, 0.9936) ccw projected
  arc A292 (-14.4672, -21.7646) -> (-14.818, -21.6706) centre (-14.7056, -21.9528) ccw projected
  arc A293 (-14.4672, -21.7646) -> (-13.3157, -22.9896) centre (-6.7902, -15.7019) ccw projected
  arc A294 (-13.3157, -22.9896) -> (-12.7173, -22.7178) centre (-23.8475, 0.9936) ccw projected
  arc A295 (-12.7173, -22.7178) -> (-12.8821, -21.0446) centre (-22.4988, -22.8365) ccw projected
  arc A296 (-12.722, -20.7187) -> (-12.8821, -21.0446) centre (-12.5835, -20.989) ccw projected
  arc A297 (-12.722, -20.7187) -> (-12.64, -20.6765) centre (-23.8475, 0.9936) ccw projected
  arc A298 (-12.2817, -20.7355) -> (-12.64, -20.6765) centre (-12.5004, -20.9462) ccw projected
  arc A299 (-12.2817, -20.7355) -> (-11.0156, -21.8418) centre (-5.2359, -13.9496) ccw projected
  arc A300 (-11.0156, -21.8418) -> (-10.4467, -21.5127) centre (-23.8475, 0.9936) ccw projected
  arc A301 (-10.4467, -21.5127) -> (-10.7747, -19.8637) centre (-20.1696, -22.5896) ccw projected
  arc A302 (-10.6474, -19.5237) -> (-10.7747, -19.8637) centre (-10.4831, -19.7791) ccw projected
  arc A303 (-10.6474, -19.5237) -> (-10.5699, -19.4736) centre (-23.8475, 0.9936) ccw projected
  arc A304 (-10.2076, -19.4973) -> (-10.5699, -19.4736) centre (-10.4046, -19.7284) ccw projected
  arc A305 (-10.2076, -19.4973) -> (-8.8391, -20.4741) centre (-3.8608, -12.0534) ccw projected
  arc A306 (-8.8391, -20.4741) -> (-8.3053, -20.0908) centre (-23.8475, 0.9936) ccw projected
  arc A307 (-8.3053, -20.0908) -> (-8.7933, -18.4819) centre (-17.8757, -22.1155) ccw projected
  arc A308 (-8.6999, -18.131) -> (-8.7933, -18.4819) centre (-8.5114, -18.3691) ccw projected
  arc A309 (-8.6999, -18.131) -> (-8.6277, -18.0736) centre (-23.8475, 0.9936) ccw projected
  arc A310 (-8.2648, -18.0616) -> (-8.6277, -18.0736) centre (-8.4382, -18.3109) ccw projected
  arc A311 (-8.2648, -18.0616) -> (-6.8072, -18.8997) centre (-2.6782, -10.0315) ccw projected
  arc A312 (-6.8072, -18.8997) -> (-6.3135, -18.4659) centre (-23.8475, 0.9936) ccw projected
  arc A313 (-6.3135, -18.4659) -> (-6.9569, -16.9125) centre (-15.6394, -21.4189) ccw projected
  arc A314 (-6.8983, -16.5542) -> (-6.9569, -16.9125) centre (-6.6873, -16.7726) ccw projected
  arc A315 (-6.8983, -16.5542) -> (-6.8321, -16.49) centre (-23.8475, 0.9936) ccw projected
  arc A316 (-6.4721, -16.4425) -> (-6.8321, -16.49) centre (-6.6203, -16.7076) ccw projected
  arc A317 (-6.4721, -16.4425) -> (-4.9394, -17.1336) centre (-1.6995, -7.9035) ccw projected
  arc A318 (-4.9394, -17.1336) -> (-4.4905, -16.6536) centre (-23.8475, 0.9936) ccw projected
  arc A319 (-4.4905, -16.6536) -> (-5.2831, -15.1708) centre (-13.4821, -20.5064) ccw projected
  arc A320 (-5.26, -14.8084) -> (-5.2831, -15.1708) centre (-5.0286, -15.0051) ccw projected
  arc A321 (-5.26, -14.8084) -> (-5.2003, -14.738) centre (-23.8475, 0.9936) ccw projected
  arc A322 (-4.8467, -14.6555) -> (-5.2003, -14.738) centre (-4.9682, -14.9338) ccw projected
  arc A323 (-4.8467, -14.6555) -> (-3.2537, -15.193) centre (-0.9341, -5.6897) ccw projected
  arc A324 (-3.2537, -15.193) -> (-2.854, -14.6713) centre (-23.8475, 0.9936) ccw projected
  arc A325 (-2.854, -14.6713) -> (-3.7881, -13.2733) centre (-11.4247, -19.3869) ccw projected
  arc A326 (-3.8006, -12.9104) -> (-3.7881, -13.2733) centre (-3.5511, -13.0835) ccw projected
  arc A327 (-3.8006, -12.9104) -> (-3.7481, -12.8345) centre (-23.8475, 0.9936) ccw projected
  arc A328 (-3.4044, -12.7177) -> (-3.7481, -12.8345) centre (-3.498, -13.0066) ccw projected
  arc A329 (-3.4044, -12.7177) -> (-1.7663, -13.0965) centre (-0.3894, -3.4117) ccw projected
  arc A330 (-1.7663, -13.0965) -> (-1.4197, -12.5381) centre (-23.8475, 0.9936) ccw projected
  arc A331 (-1.4197, -12.5381) -> (-2.4863, -11.2384) centre (-9.4868, -18.0711) ccw projected
  arc A332 (-2.5343, -10.8785) -> (-2.4863, -11.2384) centre (-2.269, -11.0263) ccw projected
  arc A333 (-2.5343, -10.8785) -> (-2.4895, -10.7978) centre (-23.8475, 0.9936) ccw projected
  arc A334 (-2.1589, -10.6479) -> (-2.4895, -10.7978) centre (-2.2237, -10.9446) ccw projected
  arc A335 (-2.1589, -10.6479) -> (-0.4915, -10.8644) centre (-0.0705, -1.0911) ccw projected
  arc A336 (-0.4915, -10.8644) -> (-0.2014, -10.2746) centre (-23.8475, 0.9936) ccw projected
  arc A337 (-0.2014, -10.2746) -> (-1.3902, -9.0858) centre (-7.6873, -16.5717) ccw projected
  arc A338 (-1.4733, -8.7323) -> (-1.3902, -9.0858) centre (-1.1947, -8.8534) ccw projected
  arc A339 (-1.4733, -8.7323) -> (-1.4366, -8.6476) centre (-23.8475, 0.9936) ccw projected
  arc A340 (-1.1222, -8.466) -> (-1.4366, -8.6476) centre (-1.1577, -8.7676) ccw projected
  arc A341 (-1.1222, -8.466) -> (0.5583, -8.518) centre (0.0193, 1.2494) ccw projected
  arc A342 (0.5583, -8.518) -> (0.7893, -7.9027) centre (-23.8475, 0.9936) ccw projected
  arc A343 (0.7893, -7.9027) -> (-0.5104, -6.836) centre (-6.0434, -14.9032) ccw projected
  arc A344 (-0.6277, -6.4924) -> (-0.5104, -6.836) centre (-0.3387, -6.5856) ccw projected
  arc A345 (-0.6277, -6.4924) -> (-0.5995, -6.4045) centre (-23.8475, 0.9936) ccw projected
  arc A346 (-0.3045, -6.193) -> (-0.5995, -6.4045) centre (-0.3102, -6.4966) ccw projected
  arc A347 (-0.3045, -6.193) -> (1.3731, -6.08) centre (-0.1207, 3.5876) ccw projected
  arc A348 (1.3731, -6.08) -> (1.5426, -5.445) centre (-23.8475, 0.9936) ccw projected
  arc A349 (1.5426, -5.445) -> (0.1446, -4.5109) centre (-4.571, -13.0815) ccw projected
  arc A350 (-0.0058, -4.1804) -> (0.1446, -4.5109) centre (0.291, -4.2448) ccw projected
  arc A351 (-0.0058, -4.1804) -> (0.0136, -4.0902) centre (-23.8475, 0.9936) ccw projected
  arc A352 (0.2866, -3.8508) -> (0.0136, -4.0902) centre (0.3107, -4.1535) ccw projected
  arc A353 (0.2866, -3.8508) -> (1.945, -3.5739) centre (-0.4892, 5.9007) ccw projected
  arc A354 (1.945, -3.5739) -> (2.0514, -2.9253) centre (-23.8475, 0.9936) ccw projected
  arc A355 (2.0514, -2.9253) -> (0.5686, -2.1328) centre (-3.2842, -11.1243) ccw projected
  arc A356 (0.3866, -1.8186) -> (0.5686, -2.1328) centre (0.6882, -1.8536) ccw projected
  arc A357 (0.3866, -1.8186) -> (0.397, -1.7269) centre (-23.8475, 0.9936) ccw projected
  arc A358 (0.6452, -1.4619) -> (0.397, -1.7269) centre (0.6988, -1.7608) ccw projected
  arc A359 (0.6452, -1.4619) -> (2.2684, -1.0238) centre (-1.0827, 8.1666) ccw projected
  arc A360 (2.2684, -1.0238) -> (2.3108, -0.3679) centre (-23.8475, 0.9936) ccw projected
  arc A361 (2.3108, -0.3679) -> (0.7575, 0.2755) centre (-2.1955, -9.0504) ccw projected
  arc A362 (0.5455, 0.5703) -> (0.7575, 0.2755) centre (0.8492, 0.565) ccw projected
  arc A363 (0.5455, 0.5703) -> (0.547, 0.6626) centre (-23.8475, 0.9936) ccw projected
  arc A364 (0.7679, 0.9507) -> (0.547, 0.6626) centre (0.8506, 0.6584) ccw projected
  arc A365 (0.7679, 0.9507) -> (2.3404, 1.5457) centre (-1.8954, 10.3634) ccw projected
  arc A366 (2.3404, 1.5457) -> (2.3183, 2.2026) centre (-23.8475, 0.9936) ccw projected
  arc A367 (2.3183, 2.2026) -> (0.7094, 2.6907) centre (-1.3153, -6.8798) ccw projected
  arc A368 (0.4696, 2.9633) -> (0.7094, 2.6907) centre (0.7722, 2.9878) ccw projected
  arc A369 (0.4696, 2.9633) -> (0.4619, 3.0552) centre (-23.8475, 0.9936) ccw projected
  arc A370 (0.6536, 3.3636) -> (0.4619, 3.0552) centre (0.7645, 3.0809) ccw projected
  arc A371 (0.6536, 3.3636) -> (2.1602, 4.11) centre (-2.9195, 12.47) ccw projected
  arc A372 (2.1602, 4.11) -> (2.0738, 4.7615) centre (-23.8475, 0.9936) ccw projected
  arc A373 (2.0738, 4.7615) -> (0.4248, 5.0895) centre (-0.6521, -4.6333) ccw projected
  arc A374 (0.1594, 5.3373) -> (0.4248, 5.0895) centre (0.4582, 5.3913) ccw projected
  arc A375 (0.1594, 5.3373) -> (0.1428, 5.428) centre (-23.8475, 0.9936) ccw projected
  arc A376 (0.3033, 5.7537) -> (0.1428, 5.428) centre (0.4414, 5.4832) ccw projected
  arc A377 (0.3033, 5.7537) -> (1.7295, 6.6441) centre (-4.1451, 14.466) ccw projected
  arc A378 (1.7295, 6.6441) -> (1.5797, 7.2841) centre (-23.8475, 0.9936) ccw projected
  arc A379 (1.5797, 7.2841) -> (-0.0936, 7.4489) centre (-0.2122, -2.3327) ccw projected
  arc A380 (-0.382, 7.6694) -> (-0.0936, 7.4489) centre (-0.0899, 7.7525) ccw projected
  arc A381 (-0.382, 7.6694) -> (-0.4074, 7.7581) centre (-23.8475, 0.9936) ccw projected
  arc A382 (-0.2795, 8.098) -> (-0.4074, 7.7581) centre (-0.1156, 7.8424) ccw projected
  arc A383 (-0.2795, 8.098) -> (1.0525, 9.1239) centre (-5.5605, 16.3323) ccw projected
  circle A384 centre (-23.8475, 0.9936) radius 4.7625 projected
  circle A385 centre (-23.8475, 0.9936) radius 28.6361 projected
extrude "Extrusion2" add sketch "Sketch2" along normal blind 4.826 contours A385
sketch "Sketch3" plane through (0, 0, 31.877) normal (0, 0, 1) x (1, 0, 0)
  circle A0 centre (0, 0) radius 28.6361 projected
  line L0 (-28.6361, 0) -> (28.6361, 0)
  line L1 (0.6848, 24.3871) -> (0.6848, 29.4671)
  circle A1 centre (0, 0) radius 29.475
  circle A2 centre (0, 0) radius 28.6361
  point P0 (0, 0)
  dimension "d5" = 57.2721
  dimension "d7" = 5.08
  constraints: 4 end point, 2 point on circle, 1 centre point, 1 coincident, 1 concentric, 1 horizontal, 1 vertical, 3 other
  measures "d5" distance of L0.start L0.end
  measures "d7" distance of L1.start L1.end
extrude "Extrusion3" add sketch "Sketch3" against normal blind 4.826